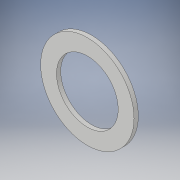
# Autodesk Inventor part: Fixierplatte_Innenring58,2mm
Saved by Autodesk Inventor 2018 (Build 220112000, 112)
## iProperties
Created: 2020-01-21
Part Number: Fixierplatte_Innenring58,2mm
Material: Generisch
Document SubType Name: Modeling
Designer: maxse
Density: 1 g/cm^3
Appearance: Vorgabe
Author: maxse
Autodesk Inventor part; units mm, degrees
ref_plane "YZ Plane" through (0, 0, 0) normal (1, 0, 0) x (0, 1, 0)
ref_plane "XZ Plane" through (0, 0, 0) normal (0, 1, 0) x (-1, 0, 0)
ref_plane "XY Plane" through (0, 0, 0) normal (0, 0, 1) x (1, 0, 0)
sketch "Skizze1" plane through (0, 0, 0) normal (0, 1, 0) x (-1, 0, 0)
  circle A0 centre (0, 0) radius 29.1
  circle A1 centre (0, 0) radius 44
  dimension "d0" = 58.2
  dimension "d1" = 88
  constraints: 2 centre point, 2 coincident
  measures "d0" diameter of A0
  measures "d1" diameter of A1
extrude "Extrusion1" add sketch "Skizze1" along normal blind 4
sketch "Skizze2" plane through (0, 4, 0) normal (0, 1, 0) x (1, 0, 0)
  circle A0 centre (0, 0) radius 29.1 projected
  line L0 (9.4434, -32.7819) -> (9.8648, -32.6469)
  line L1 (9.8648, -32.6469) -> (9.9461, -32.9008)
  spline S0 degree 2 poles (9.9461, -32.9008) (10.0174, -32.7886) (10.1259, -32.6347) (10.2084, -32.5576) knots 0 0 0 1 2 2 2
  spline S1 degree 2 poles (10.2084, -32.5576) (10.2837, -32.4858) (10.4608, -32.3785) (10.5877, -32.3378) knots 0 0 0 1 2 2 2
  spline S2 degree 2 poles (10.5877, -32.3378) (10.793, -32.272) (11.1933, -32.3314) (11.3676, -32.4572) knots 0 0 0 1 2 2 2
  spline S3 degree 2 poles (11.3676, -32.4572) (11.542, -32.583) (11.8328, -33.026) (11.934, -33.342) knots 0 0 0 1 2 2 2
  spline S4 degree 2 poles (11.934, -33.342) (12.0396, -33.6715) (12.0235, -34.2068) (11.9329, -34.4354) knots 0 0 0 1 2 2 2
  spline S5 degree 2 poles (11.9329, -34.4354) (11.8471, -34.6416) (11.5206, -34.9517) (11.3072, -35.0201) knots 0 0 0 1 2 2 2
  spline S6 degree 2 poles (11.3072, -35.0201) (11.1208, -35.0798) (10.8158, -35.0852) (10.6341, -35.0481) knots 0 0 0 1 2 2 2
  line L2 (10.6341, -35.0481) -> (10.9803, -36.1285)
  line L3 (10.9803, -36.1285) -> (10.559, -36.2635)
  line L4 (10.559, -36.2635) -> (9.4434, -32.7819)
  line L5 (10.0595, -33.2546) -> (10.5225, -34.6997)
  spline S7 degree 2 poles (10.5225, -34.6997) (10.7034, -34.7251) (10.9701, -34.7022) (11.1132, -34.6563) knots 0 0 0 1 2 2 2
  spline S8 degree 2 poles (11.1132, -34.6563) (11.4373, -34.5525) (11.6489, -33.9486) (11.5018, -33.4894) knots 0 0 0 1 2 2 2
  spline S9 degree 2 poles (11.5018, -33.4894) (11.3598, -33.0464) (10.9292, -32.6692) (10.6186, -32.7687) knots 0 0 0 1 2 2 2
  spline S10 degree 2 poles (10.6186, -32.7687) (10.4538, -32.8215) (10.1674, -33.0801) (10.0595, -33.2546) knots 0 0 0 1 2 2 2
  spline S11 degree 2 poles (7.7028, -33.158) (8.3153, -33.0121) (9.1523, -33.5386) (9.3035, -34.1732) knots 0 0 0 1 2 2 2
  spline S12 degree 2 poles (9.3035, -34.1732) (9.4521, -34.7967) (8.9744, -35.692) (8.4475, -35.8176) knots 0 0 0 1 2 2 2
  spline S13 degree 2 poles (8.4475, -35.8176) (8.2102, -35.8741) (7.8104, -35.8236) (7.6403, -35.7096) knots 0 0 0 1 2 2 2
  spline S14 degree 2 poles (7.6403, -35.7096) (7.4675, -35.5963) (7.2207, -35.209) (7.1477, -34.9028) knots 0 0 0 1 2 2 2
  line L6 (7.1477, -34.9028) -> (7.0918, -34.6682)
  line L7 (7.0918, -34.6682) -> (8.8603, -34.2467)
  spline S15 degree 2 poles (8.8603, -34.2467) (8.7545, -33.8025) (8.1951, -33.4373) (7.7978, -33.532) knots 0 0 0 1 2 2 2
  spline S16 degree 2 poles (7.7978, -33.532) (7.6571, -33.5655) (7.399, -33.694) (7.3005, -33.77) knots 0 0 0 1 2 2 2
  spline S17 degree 2 poles (7.3005, -33.77) (7.1978, -33.8528) (7.0608, -33.9875) (7.0189, -34.0442) knots 0 0 0 1 2 2 2
  line L8 (7.0189, -34.0442) -> (6.994, -34.0501)
  line L9 (6.994, -34.0501) -> (6.8823, -33.581)
  spline S18 degree 2 poles (6.8823, -33.581) (6.9495, -33.5329) (7.1547, -33.3907) (7.2371, -33.3448) knots 0 0 0 1 2 2 2
  spline S19 degree 2 poles (7.2371, -33.3448) (7.3527, -33.2794) (7.5483, -33.1949) (7.7028, -33.158) knots 0 0 0 1 2 2 2
  spline S20 degree 2 poles (7.5894, -34.8966) (7.6364, -35.0691) (7.7686, -35.3058) (7.858, -35.3749) knots 0 0 0 1 2 2 2
  spline S21 degree 2 poles (7.858, -35.3749) (7.9555, -35.4537) (8.2143, -35.4999) (8.3881, -35.4585) knots 0 0 0 1 2 2 2
  spline S22 degree 2 poles (8.3881, -35.4585) (8.5592, -35.4177) (8.7749, -35.2585) (8.8506, -35.1355) knots 0 0 0 1 2 2 2
  spline S23 degree 2 poles (8.8506, -35.1355) (8.9228, -35.0104) (8.9636, -34.7411) (8.9386, -34.5751) knots 0 0 0 1 2 2 2
  line L10 (8.9386, -34.5751) -> (7.5894, -34.8966)
  spline S24 degree 2 poles (5.6466, -33.566) (5.9068, -33.5226) (6.3806, -33.5873) (6.5419, -33.6409) knots 0 0 0 1 2 2 2
  line L11 (6.5419, -33.6409) -> (6.6236, -34.1304)
  line L12 (6.6236, -34.1304) -> (6.6012, -34.1342)
  spline S25 degree 2 poles (6.6012, -34.1342) (6.5378, -34.0988) (6.369, -34.0177) (6.2333, -33.9799) knots 0 0 0 1 2 2 2
  spline S26 degree 2 poles (6.2333, -33.9799) (6.1153, -33.945) (5.8337, -33.9115) (5.691, -33.9353) knots 0 0 0 1 2 2 2
  spline S27 degree 2 poles (5.691, -33.9353) (5.5875, -33.9526) (5.3576, -34.0398) (5.3082, -34.0883) knots 0 0 0 1 2 2 2
  spline S28 degree 2 poles (5.3082, -34.0883) (5.236, -34.155) (5.1833, -34.2874) (5.2038, -34.4105) knots 0 0 0 1 2 2 2
  spline S29 degree 2 poles (5.2038, -34.4105) (5.2295, -34.5644) (5.424, -34.6959) (5.6483, -34.7131) knots 0 0 0 1 2 2 2
  spline S30 degree 2 poles (5.6483, -34.7131) (5.7355, -34.7186) (6.0134, -34.7298) (6.1332, -34.7414) knots 0 0 0 1 2 2 2
  spline S31 degree 2 poles (6.1332, -34.7414) (6.4442, -34.7786) (6.7726, -35.0919) (6.8151, -35.3465) knots 0 0 0 1 2 2 2
  spline S32 degree 2 poles (6.8151, -35.3465) (6.8739, -35.699) (6.4185, -36.2264) (5.982, -36.2993) knots 0 0 0 1 2 2 2
  spline S33 degree 2 poles (5.982, -36.2993) (5.7666, -36.3352) (5.3124, -36.3018) (5.1506, -36.2454) knots 0 0 0 1 2 2 2
  line L13 (5.1506, -36.2454) -> (5.0726, -35.7782)
  line L14 (5.0726, -35.7782) -> (5.095, -35.7744)
  spline S34 degree 2 poles (5.095, -35.7744) (5.2853, -35.8807) (5.7194, -35.9664) (5.9293, -35.9314) knots 0 0 0 1 2 2 2
  spline S35 degree 2 poles (5.9293, -35.9314) (6.1447, -35.8954) (6.4109, -35.6641) (6.3805, -35.4823) knots 0 0 0 1 2 2 2
  spline S36 degree 2 poles (6.3805, -35.4823) (6.353, -35.3172) (6.1501, -35.1872) (5.9459, -35.1695) knots 0 0 0 1 2 2 2
  spline S37 degree 2 poles (5.9459, -35.1695) (5.8465, -35.1602) (5.5975, -35.15) (5.4609, -35.1411) knots 0 0 0 1 2 2 2
  spline S38 degree 2 poles (5.4609, -35.1411) (5.1634, -35.116) (4.8169, -34.8317) (4.7688, -34.5435) knots 0 0 0 1 2 2 2
  spline S39 degree 2 poles (4.7688, -34.5435) (4.7408, -34.3757) (4.8228, -34.0572) (4.9333, -33.9266) knots 0 0 0 1 2 2 2
  spline S40 degree 2 poles (4.9333, -33.9266) (5.0512, -33.789) (5.3808, -33.6104) (5.6466, -33.566) knots 0 0 0 1 2 2 2
  line L15 (3.7868, -33.8898) -> (4.2262, -33.8378)
  line L16 (4.2262, -33.8378) -> (4.5348, -36.446)
  line L17 (4.5348, -36.446) -> (4.0954, -36.498)
  line L18 (4.0954, -36.498) -> (3.7868, -33.8898)
  line L19 (4.1158, -36.9355) -> (4.6143, -36.8765)
  line L20 (4.6143, -36.8765) -> (4.6683, -37.3328)
  line L21 (4.6683, -37.3328) -> (4.1697, -37.3918)
  line L22 (4.1697, -37.3918) -> (4.1158, -36.9355)
  spline S41 degree 2 poles (3.0227, -33.5568) (2.9762, -33.5398) (2.7996, -33.4884) (2.6876, -33.4698) knots 0 0 0 1 2 2 2
  spline S42 degree 2 poles (2.6876, -33.4698) (2.5639, -33.4463) (2.355, -33.4225) (2.2333, -33.4301) knots 0 0 0 1 2 2 2
  spline S43 degree 2 poles (2.2333, -33.4301) (2.0294, -33.4429) (1.7531, -33.5682) (1.6799, -33.6695) knots 0 0 0 1 2 2 2
  spline S44 degree 2 poles (1.6799, -33.6695) (1.6095, -33.7705) (1.5659, -34.0262) (1.576, -34.1875) knots 0 0 0 1 2 2 2
  line L23 (1.576, -34.1875) -> (1.5904, -34.4168)
  spline S45 degree 2 poles (1.5904, -34.4168) (1.7589, -34.2499) (2.0922, -34.0813) (2.3498, -34.0651) knots 0 0 0 1 2 2 2
  spline S46 degree 2 poles (2.3498, -34.0651) (2.7971, -34.037) (3.3681, -34.6691) (3.4074, -35.2947) knots 0 0 0 1 2 2 2
  spline S47 degree 2 poles (3.4074, -35.2947) (3.4278, -35.6202) (3.2754, -36.1356) (3.1337, -36.3235) knots 0 0 0 1 2 2 2
  spline S48 degree 2 poles (3.1337, -36.3235) (2.997, -36.4998) (2.6038, -36.7092) (2.3886, -36.7227) knots 0 0 0 1 2 2 2
  spline S49 degree 2 poles (2.3886, -36.7227) (2.1848, -36.7354) (1.8815, -36.6578) (1.726, -36.5795) knots 0 0 0 1 2 2 2
  line L24 (1.726, -36.5795) -> (1.7075, -36.6915)
  line L25 (1.7075, -36.6915) -> (1.2913, -36.7176)
  line L26 (1.2913, -36.7176) -> (1.1457, -34.3964)
  spline S50 degree 2 poles (1.1457, -34.3964) (1.1038, -33.7283) (1.6451, -33.0692) (2.2424, -33.0317) knots 0 0 0 1 2 2 2
  spline S51 degree 2 poles (2.2424, -33.0317) (2.4349, -33.0196) (2.8407, -33.0567) (3.0166, -33.0968) knots 0 0 0 1 2 2 2
  line L27 (3.0166, -33.0968) -> (3.0454, -33.5554)
  line L28 (3.0454, -33.5554) -> (3.0227, -33.5568)
  line L29 (1.6131, -34.7791) -> (1.7035, -36.22)
  spline S52 degree 2 poles (1.7035, -36.22) (1.8726, -36.289) (2.1543, -36.3395) (2.293, -36.3308) knots 0 0 0 1 2 2 2
  spline S53 degree 2 poles (2.293, -36.3308) (2.627, -36.3098) (2.9811, -35.7931) (2.9522, -35.3317) knots 0 0 0 1 2 2 2
  spline S54 degree 2 poles (2.9522, -35.3317) (2.9248, -34.8958) (2.6047, -34.4583) (2.2763, -34.4789) knots 0 0 0 1 2 2 2
  spline S55 degree 2 poles (2.2763, -34.4789) (2.1036, -34.4898) (1.7498, -34.6484) (1.6131, -34.7791) knots 0 0 0 1 2 2 2
  line L30 (-1.5751, -34.0795) -> (-1.1327, -34.0864)
  line L31 (-1.1327, -34.0864) -> (-1.1562, -35.5838)
  spline S56 degree 2 poles (-1.1562, -35.5838) (-1.159, -35.7653) (-1.1299, -36.0778) (-1.0803, -36.1722) knots 0 0 0 1 2 2 2
  spline S57 degree 2 poles (-1.0803, -36.1722) (-1.028, -36.2723) (-0.8367, -36.3717) (-0.6722, -36.3743) knots 0 0 0 1 2 2 2
  spline S58 degree 2 poles (-0.6722, -36.3743) (-0.5077, -36.3769) (-0.1561, -36.2065) (0.0134, -36.0674) knots 0 0 0 1 2 2 2
  line L32 (0.0134, -36.0674) -> (0.0442, -34.1049)
  line L33 (0.0442, -34.1049) -> (0.4866, -34.1118)
  line L34 (0.4866, -34.1118) -> (0.4454, -36.7379)
  line L35 (0.4454, -36.7379) -> (0.003, -36.731)
  line L36 (0.003, -36.731) -> (0.0076, -36.4389)
  spline S59 degree 2 poles (0.0076, -36.4389) (-0.1937, -36.6144) (-0.5795, -36.7956) (-0.795, -36.7922) knots 0 0 0 1 2 2 2
  spline S60 degree 2 poles (-0.795, -36.7922) (-1.1807, -36.7862) (-1.6095, -36.2689) (-1.6019, -35.7839) knots 0 0 0 1 2 2 2
  line L37 (-1.6019, -35.7839) -> (-1.5751, -34.0795)
  spline S61 degree 2 poles (-3.3246, -33.8783) (-2.6976, -33.9362) (-2.0735, -34.7031) (-2.1335, -35.3527) knots 0 0 0 1 2 2 2
  spline S62 degree 2 poles (-2.1335, -35.3527) (-2.1924, -35.9909) (-2.9317, -36.686) (-3.4711, -36.6362) knots 0 0 0 1 2 2 2
  spline S63 degree 2 poles (-3.4711, -36.6362) (-3.714, -36.6138) (-4.0766, -36.4378) (-4.2012, -36.2754) knots 0 0 0 1 2 2 2
  spline S64 degree 2 poles (-4.2012, -36.2754) (-4.3286, -36.1126) (-4.4383, -35.6667) (-4.4094, -35.3532) knots 0 0 0 1 2 2 2
  line L38 (-4.4094, -35.3532) -> (-4.3872, -35.1131)
  line L39 (-4.3872, -35.1131) -> (-2.5768, -35.2804)
  spline S65 degree 2 poles (-2.5768, -35.2804) (-2.5348, -34.8257) (-2.9478, -34.3004) (-3.3545, -34.2629) knots 0 0 0 1 2 2 2
  spline S66 degree 2 poles (-3.3545, -34.2629) (-3.4985, -34.2496) (-3.7841, -34.2887) (-3.9018, -34.3291) knots 0 0 0 1 2 2 2
  spline S67 degree 2 poles (-3.9018, -34.3291) (-4.0256, -34.3746) (-4.1985, -34.4583) (-4.2564, -34.4986) knots 0 0 0 1 2 2 2
  line L40 (-4.2564, -34.4986) -> (-4.2818, -34.4962)
  line L41 (-4.2818, -34.4962) -> (-4.2374, -34.0161)
  spline S68 degree 2 poles (-4.2374, -34.0161) (-4.1583, -33.9921) (-3.9184, -33.9231) (-3.8257, -33.906) knots 0 0 0 1 2 2 2
  spline S69 degree 2 poles (-3.8257, -33.906) (-3.6952, -33.8811) (-3.4828, -33.8636) (-3.3246, -33.8783) knots 0 0 0 1 2 2 2
  spline S70 degree 2 poles (-3.989, -35.4889) (-3.9997, -35.6673) (-3.9503, -35.934) (-3.8878, -36.028) knots 0 0 0 1 2 2 2
  spline S71 degree 2 poles (-3.8878, -36.028) (-3.8207, -36.1339) (-3.5903, -36.2606) (-3.4123, -36.277) knots 0 0 0 1 2 2 2
  spline S72 degree 2 poles (-3.4123, -36.277) (-3.2372, -36.2932) (-2.9819, -36.2114) (-2.8708, -36.1191) knots 0 0 0 1 2 2 2
  spline S73 degree 2 poles (-2.8708, -36.1191) (-2.7623, -36.0238) (-2.6374, -35.7818) (-2.6079, -35.6165) knots 0 0 0 1 2 2 2
  line L42 (-2.6079, -35.6165) -> (-3.989, -35.4889)
  line L43 (-6.7049, -33.4496) -> (-6.2687, -33.5237)
  line L44 (-6.2687, -33.5237) -> (-6.3133, -33.7865)
  spline S74 degree 2 poles (-6.3133, -33.7865) (-6.1984, -33.7197) (-6.0312, -33.633) (-5.9225, -33.6026) knots 0 0 0 1 2 2 2
  spline S75 degree 2 poles (-5.9225, -33.6026) (-5.8226, -33.5735) (-5.616, -33.5597) (-5.4846, -33.582) knots 0 0 0 1 2 2 2
  spline S76 degree 2 poles (-5.4846, -33.582) (-5.2721, -33.6181) (-4.9441, -33.8551) (-4.8472, -34.047) knots 0 0 0 1 2 2 2
  spline S77 degree 2 poles (-4.8472, -34.047) (-4.7503, -34.2389) (-4.696, -34.766) (-4.7516, -35.0932) knots 0 0 0 1 2 2 2
  spline S78 degree 2 poles (-4.7516, -35.0932) (-4.8095, -35.4343) (-5.0702, -35.9021) (-5.2558, -36.0634) knots 0 0 0 1 2 2 2
  spline S79 degree 2 poles (-5.2558, -36.0634) (-5.4269, -36.2069) (-5.8595, -36.332) (-6.0804, -36.2944) knots 0 0 0 1 2 2 2
  spline S80 degree 2 poles (-6.0804, -36.2944) (-6.2734, -36.2617) (-6.5467, -36.1261) (-6.6909, -36.0095) knots 0 0 0 1 2 2 2
  line L45 (-6.6909, -36.0095) -> (-6.8808, -37.128)
  line L46 (-6.8808, -37.128) -> (-7.317, -37.054)
  line L47 (-7.317, -37.054) -> (-6.7049, -33.4496)
  line L48 (-6.3755, -34.1528) -> (-6.6296, -35.6488)
  spline S81 degree 2 poles (-6.6296, -35.6488) (-6.4807, -35.7547) (-6.2334, -35.8571) (-6.0852, -35.8822) knots 0 0 0 1 2 2 2
  spline S82 degree 2 poles (-6.0852, -35.8822) (-5.7497, -35.9392) (-5.2839, -35.5005) (-5.2032, -35.0251) knots 0 0 0 1 2 2 2
  spline S83 degree 2 poles (-5.2032, -35.0251) (-5.1253, -34.5665) (-5.334, -34.0334) (-5.6555, -33.9788) knots 0 0 0 1 2 2 2
  spline S84 degree 2 poles (-5.6555, -33.9788) (-5.8261, -33.9498) (-6.1994, -34.0475) (-6.3755, -34.1528) knots 0 0 0 1 2 2 2
  spline S85 degree 2 poles (-11.2896, -33.6315) (-11.1053, -33.0145) (-10.2826, -32.4404) (-9.8314, -32.5751) knots 0 0 0 1 2 2 2
  spline S86 degree 2 poles (-9.8314, -32.5751) (-9.6276, -32.636) (-9.3669, -32.8234) (-9.2515, -32.9526) knots 0 0 0 1 2 2 2
  line L49 (-9.2515, -32.9526) -> (-9.1894, -32.8439)
  line L50 (-9.1894, -32.8439) -> (-8.7927, -32.9624)
  line L51 (-8.7927, -32.9624) -> (-9.8391, -36.4654)
  line L52 (-9.8391, -36.4654) -> (-10.263, -36.3388)
  line L53 (-10.263, -36.3388) -> (-9.8896, -35.0887)
  spline S87 degree 2 poles (-9.8896, -35.0887) (-10.093, -35.1848) (-10.5221, -35.2638) (-10.7585, -35.1932) knots 0 0 0 1 2 2 2
  spline S88 degree 2 poles (-10.7585, -35.1932) (-11.1852, -35.0657) (-11.4706, -34.2375) (-11.2896, -33.6315) knots 0 0 0 1 2 2 2
  spline S89 degree 2 poles (-10.8423, -33.7295) (-10.9771, -34.1807) (-10.8422, -34.7301) (-10.5378, -34.821) knots 0 0 0 1 2 2 2
  spline S90 degree 2 poles (-10.5378, -34.821) (-10.3666, -34.8722) (-9.9646, -34.8146) (-9.7832, -34.7327) knots 0 0 0 1 2 2 2
  line L54 (-9.7832, -34.7327) -> (-9.3522, -33.2896)
  spline S91 degree 2 poles (-9.3522, -33.2896) (-9.489, -33.1629) (-9.7168, -33.0238) (-9.8635, -32.9799) knots 0 0 0 1 2 2 2
  spline S92 degree 2 poles (-9.8635, -32.9799) (-10.1869, -32.8833) (-10.6937, -33.2322) (-10.8423, -33.7295) knots 0 0 0 1 2 2 2
  line L55 (-14.1952, -33.8929) -> (-11.5948, -31.0386)
  line L56 (-11.5948, -31.0386) -> (-11.1522, -31.2075)
  line L57 (-11.1522, -31.2075) -> (-11.9823, -32.0626)
  line L58 (-11.9823, -32.0626) -> (-11.9824, -34.7369)
  line L59 (-11.9824, -34.7369) -> (-12.4276, -34.5671)
  line L60 (-12.4276, -34.5671) -> (-12.4047, -32.4934)
  line L61 (-12.4047, -32.4934) -> (-13.7659, -34.0566)
  line L62 (-13.7659, -34.0566) -> (-14.1952, -33.8929)
  line L63 (18.0086, 34.7463) -> (16.5324, 31.5728)
  line L64 (16.5324, 31.5728) -> (15.9011, 31.8665)
  line L65 (15.9011, 31.8665) -> (16.1941, 34.4634)
  spline S93 degree 2 poles (16.1941, 34.4634) (16.2363, 34.8263) (16.26, 35.0036) knots 0 0 0 1 1 1
  spline S94 degree 2 poles (16.26, 35.0036) (16.1269, 34.8566) (15.8544, 34.5744) knots 0 0 0 1 1 1
  line L66 (15.8544, 34.5744) -> (14.0652, 32.7204)
  line L67 (14.0652, 32.7204) -> (13.5016, 32.9826)
  line L68 (13.5016, 32.9826) -> (14.9778, 36.1561)
  line L69 (14.9778, 36.1561) -> (15.3817, 35.9682)
  line L70 (15.3817, 35.9682) -> (14.1463, 33.3123)
  line L71 (14.1463, 33.3123) -> (16.3081, 35.5372)
  line L72 (16.3081, 35.5372) -> (16.6855, 35.3617)
  line L73 (16.6855, 35.3617) -> (16.3479, 32.2324)
  line L74 (16.3479, 32.2324) -> (17.6046, 34.9342)
  line L75 (17.6046, 34.9342) -> (18.0086, 34.7463)
  spline S95 degree 2 poles (12.6685, 36.6659) (12.9634, 36.7745) (13.4336, 36.7796) (13.6718, 36.693) knots 0 0 0 1 2 2 2
  spline S96 degree 2 poles (13.6718, 36.693) (14.0654, 36.5499) (14.3472, 36.0132) (14.2388, 35.7149) knots 0 0 0 1 2 2 2
  spline S97 degree 2 poles (14.2388, 35.7149) (14.175, 35.5394) (13.9098, 35.3094) (13.5902, 35.2268) (13.4118, 35.2434) knots 0 0 0 1 2 3 3 3
  spline S98 degree 2 poles (13.4118, 35.2434) (13.2821, 35.2536) (13.0305, 35.311) knots 0 0 0 1 1 1
  spline S99 degree 2 poles (13.0305, 35.311) (12.5206, 35.431) (12.2608, 35.4346) knots 0 0 0 1 1 1
  spline S100 degree 2 poles (12.2608, 35.4346) (12.2282, 35.3528) (12.22, 35.3303) knots 0 0 0 1 1 1
  spline S101 degree 2 poles (12.22, 35.3303) (12.1298, 35.082) (12.2087, 34.9398) knots 0 0 0 1 1 1
  spline S102 degree 2 poles (12.2087, 34.9398) (12.3115, 34.7464) (12.6174, 34.6352) knots 0 0 0 1 1 1
  spline S103 degree 2 poles (12.6174, 34.6352) (12.9007, 34.5322) (13.2444, 34.6344) (13.4016, 34.8639) knots 0 0 0 1 2 2 2
  line L76 (13.4016, 34.8639) -> (13.7786, 34.6673)
  spline S104 degree 2 poles (13.7786, 34.6673) (13.6339, 34.4332) (13.2718, 34.21) (12.7444, 34.2115) (12.4385, 34.3227) knots 0 0 0 1 2 3 3 3
  spline S105 degree 2 poles (12.4385, 34.3227) (12.1326, 34.4338) (11.8035, 34.7153) (11.7022, 34.999) (11.7273, 35.1772) knots 0 0 0 1 2 3 3 3
  spline S106 degree 2 poles (11.7273, 35.1772) (11.7455, 35.2898) (11.843, 35.5581) knots 0 0 0 1 1 1
  line L77 (11.843, 35.5581) -> (12.0389, 36.0972)
  spline S107 degree 2 poles (12.0389, 36.0972) (12.243, 36.6588) (12.2988, 36.9763) (12.2737, 37.1415) knots 0 0 0 1 2 2 2
  line L78 (12.2737, 37.1415) -> (12.6949, 36.9884)
  spline S108 degree 2 poles (12.6949, 36.9884) (12.712, 36.8403) (12.6685, 36.6659) knots 0 0 0 1 1 1
  spline S109 degree 2 poles (12.3731, 35.7515) (12.6265, 35.7615) (13.0881, 35.6648) knots 0 0 0 1 1 1
  spline S110 degree 2 poles (13.0881, 35.6648) (13.3515, 35.6087) (13.5899, 35.6243) (13.7656, 35.7563) (13.8039, 35.8616) knots 0 0 0 1 2 3 3 3
  spline S111 degree 2 poles (13.8039, 35.8616) (13.8622, 36.022) (13.6974, 36.3261) (13.4617, 36.4117) knots 0 0 0 1 2 2 2
  spline S112 degree 2 poles (13.4617, 36.4117) (13.2285, 36.4965) (12.7912, 36.4255) (12.6412, 36.2785) knots 0 0 0 1 2 2 2
  spline S113 degree 2 poles (12.6412, 36.2785) (12.5259, 36.1643) (12.4293, 35.8985) knots 0 0 0 1 1 1
  line L79 (12.4293, 35.8985) -> (12.3731, 35.7515)
  line L80 (12.0434, 37.218) -> (10.7859, 36.2164)
  line L81 (10.7859, 36.2164) -> (11.2694, 34.801)
  line L82 (11.2694, 34.801) -> (10.7571, 34.9497)
  line L83 (10.7571, 34.9497) -> (10.5438, 35.6311)
  spline S114 degree 2 poles (10.5438, 35.6311) (10.483, 35.8238) (10.4502, 35.95) knots 0 0 0 1 1 1
  spline S115 degree 2 poles (10.4502, 35.95) (10.3061, 35.8362) (10.1899, 35.7422) knots 0 0 0 1 1 1
  line L84 (10.1899, 35.7422) -> (9.6119, 35.2822)
  line L85 (9.6119, 35.2822) -> (9.1149, 35.4265)
  line L86 (9.1149, 35.4265) -> (10.279, 36.3552)
  line L87 (10.279, 36.3552) -> (9.7633, 37.88)
  line L88 (9.7633, 37.88) -> (10.2706, 37.7327)
  line L89 (10.2706, 37.7327) -> (10.554, 36.8337)
  line L90 (10.554, 36.8337) -> (10.6183, 36.6151)
  line L91 (10.6183, 36.6151) -> (11.5439, 37.363)
  line L92 (11.5439, 37.363) -> (12.0434, 37.218)
  line L93 (7.9981, 37.1493) -> (7.5608, 37.1886)
  spline S116 degree 2 poles (7.5608, 37.1886) (7.5752, 37.4543) (7.4104, 37.8247) (6.9763, 38.1127) (6.6821, 38.1647) knots 0 0 0 1 2 3 3 3
  spline S117 degree 2 poles (6.6821, 38.1647) (6.4221, 38.2106) (5.9927, 38.1267) (5.7505, 37.8904) (5.7222, 37.7302) knots 0 0 0 1 2 3 3 3
  spline S118 degree 2 poles (5.7222, 37.7302) (5.6934, 37.5673) (5.8373, 37.2927) (6.0409, 37.1727) knots 0 0 0 1 2 2 2
  spline S119 degree 2 poles (6.0409, 37.1727) (6.1704, 37.0929) (7.0836, 36.6959) (7.2573, 36.5596) knots 0 0 0 1 2 2 2
  spline S120 degree 2 poles (7.2573, 36.5596) (7.4815, 36.3872) (7.6554, 35.961) (7.6136, 35.7245) knots 0 0 0 1 2 2 2
  spline S121 degree 2 poles (7.6136, 35.7245) (7.5672, 35.4618) (7.1905, 35.0625) (6.5787, 34.9267) (6.2293, 34.9885) knots 0 0 0 1 2 3 3 3
  spline S122 degree 2 poles (6.2293, 34.9885) (5.8458, 35.0562) (5.3036, 35.4067) (5.0706, 35.9436) (5.1135, 36.2475) knots 0 0 0 1 2 3 3 3
  line L94 (5.1135, 36.2475) -> (5.5556, 36.2046)
  spline S123 degree 2 poles (5.5556, 36.2046) (5.5318, 35.8702) (5.8826, 35.4642) (6.2819, 35.3937) knots 0 0 0 1 2 2 2
  spline S124 degree 2 poles (6.2819, 35.3937) (6.697, 35.3203) (7.1317, 35.5577) (7.1693, 35.7705) knots 0 0 0 1 2 2 2
  spline S125 degree 2 poles (7.1693, 35.7705) (7.2023, 35.957) (7.0897, 36.1016) knots 0 0 0 1 1 1
  spline S126 degree 2 poles (7.0897, 36.1016) (6.9766, 36.2434) (5.9047, 36.6929) (5.7138, 36.8241) knots 0 0 0 1 2 2 2
  spline S127 degree 2 poles (5.7138, 36.8241) (5.439, 37.0163) (5.2278, 37.4925) (5.2765, 37.7683) knots 0 0 0 1 2 2 2
  spline S128 degree 2 poles (5.2765, 37.7683) (5.3253, 38.0441) (5.7264, 38.4744) (6.3653, 38.6406) (6.7331, 38.5756) knots 0 0 0 1 2 3 3 3
  spline S129 degree 2 poles (6.7331, 38.5756) (7.2033, 38.4925) (7.7855, 38.1079) (8.0488, 37.4979) (7.9981, 37.1493) knots 0 0 0 1 2 3 3 3
  line L95 (3.0679, 38.1643) -> (2.63, 38.2638)
  spline S130 degree 2 poles (2.63, 38.2638) (2.7745, 38.6409) (3.3822, 39.0125) (3.8202, 38.9692) knots 0 0 0 1 2 2 2
  spline S131 degree 2 poles (3.8202, 38.9692) (4.375, 38.9144) (4.9554, 38.1682) (4.8949, 37.5549) knots 0 0 0 1 2 2 2
  spline S132 degree 2 poles (4.8949, 37.5549) (4.832, 36.9178) (4.1068, 36.279) (3.5838, 36.3307) knots 0 0 0 1 2 2 2
  spline S133 degree 2 poles (3.5838, 36.3307) (3.0794, 36.3805) (2.5051, 37.1342) (2.5667, 37.7581) knots 0 0 0 1 2 2 2
  spline S134 degree 2 poles (2.5667, 37.7581) (2.5703, 37.7952) (2.5806, 37.8719) knots 0 0 0 1 1 1
  line L96 (2.5806, 37.8719) -> (4.4628, 37.6861)
  spline S135 degree 2 poles (4.4628, 37.6861) (4.4801, 38.1052) (4.1015, 38.5876) (3.7856, 38.6188) knots 0 0 0 1 2 2 2
  spline S136 degree 2 poles (3.7856, 38.6188) (3.5493, 38.6421) (3.1928, 38.4254) (3.0679, 38.1643) knots 0 0 0 1 2 2 2
  line L97 (4.4043, 37.338) -> (2.9947, 37.4772)
  spline S137 degree 2 poles (2.9947, 37.4772) (2.9924, 37.1558) (3.1091, 36.9807) knots 0 0 0 1 1 1
  spline S138 degree 2 poles (3.1091, 36.9807) (3.2892, 36.7136) (3.6157, 36.6814) knots 0 0 0 1 1 1
  spline S139 degree 2 poles (3.6157, 36.6814) (3.9104, 36.6523) (4.3503, 37.0082) (4.4043, 37.338) knots 0 0 0 1 2 2 2
  line L98 (2.3158, 38.2874) -> (1.8897, 38.2345)
  spline S140 degree 2 poles (1.8897, 38.2345) (1.8634, 38.4916) (1.5442, 38.7742) (1.2483, 38.7838) knots 0 0 0 1 2 2 2
  spline S141 degree 2 poles (1.2483, 38.7838) (0.9523, 38.7934) (0.6565, 38.5601) (0.6512, 38.3975) knots 0 0 0 1 2 2 2
  spline S142 degree 2 poles (0.6512, 38.3975) (0.6465, 38.2535) (0.7717, 38.164) knots 0 0 0 1 1 1
  spline S143 degree 2 poles (0.7717, 38.164) (0.8579, 38.1052) (1.207, 38.0058) knots 0 0 0 1 1 1
  spline S144 degree 2 poles (1.207, 38.0058) (1.6751, 37.8705) (2.0347, 37.6853) (2.214, 37.3699) (2.208, 37.1859) knots 0 0 0 1 2 3 3 3
  spline S145 degree 2 poles (2.208, 37.1859) (2.2025, 37.0153) (2.0385, 36.7323) (1.9021, 36.6407) knots 0 0 0 1 2 2 2
  spline S146 degree 2 poles (1.9021, 36.6407) (1.7984, 36.5693) (1.4484, 36.4792) (1.2485, 36.4857) knots 0 0 0 1 2 2 2
  spline S147 degree 2 poles (1.2485, 36.4857) (0.9499, 36.4954) (0.5049, 36.6833) (0.2984, 36.9836) (0.2664, 37.2302) knots 0 0 0 1 2 3 3 3
  line L99 (0.2664, 37.2302) -> (0.6895, 37.2725)
  spline S148 degree 2 poles (0.6895, 37.2725) (0.7124, 37.0743) (0.9799, 36.8467) (1.2306, 36.8386) knots 0 0 0 1 2 2 2
  spline S149 degree 2 poles (1.2306, 36.8386) (1.5265, 36.829) (1.7862, 37.0181) (1.7904, 37.1488) knots 0 0 0 1 2 2 2
  spline S150 degree 2 poles (1.7904, 37.1488) (1.7931, 37.2314) (1.742, 37.2998) knots 0 0 0 1 1 1
  spline S151 degree 2 poles (1.742, 37.2998) (1.6936, 37.3708) (1.5804, 37.4198) knots 0 0 0 1 1 1
  spline S152 degree 2 poles (1.5804, 37.4198) (1.5172, 37.4459) (1.2054, 37.5441) knots 0 0 0 1 1 1
  spline S153 degree 2 poles (1.2054, 37.5441) (0.7533, 37.6788) (0.3957, 37.8452) (0.2, 38.1479) (0.2072, 38.3692) knots 0 0 0 1 2 3 3 3
  spline S154 degree 2 poles (0.2072, 38.3692) (0.2141, 38.5825) (0.477, 38.9529) (0.9584, 39.1455) (1.257, 39.1358) knots 0 0 0 1 2 3 3 3
  spline S155 degree 2 poles (1.257, 39.1358) (1.7503, 39.1198) (2.2569, 38.6924) (2.3158, 38.2874) knots 0 0 0 1 2 2 2
  line L100 (-0.0818, 38.3573) -> (-0.5038, 38.2779)
  spline S156 degree 2 poles (-0.5038, 38.2779) (-0.5461, 38.5328) (-0.8823, 38.7949) (-1.1783, 38.786) knots 0 0 0 1 2 2 2
  spline S157 degree 2 poles (-1.1783, 38.786) (-1.4743, 38.7771) (-1.7549, 38.5257) (-1.75, 38.3631) knots 0 0 0 1 2 2 2
  spline S158 degree 2 poles (-1.75, 38.3631) (-1.7457, 38.2191) (-1.6151, 38.1376) knots 0 0 0 1 1 1
  spline S159 degree 2 poles (-1.6151, 38.1376) (-1.5254, 38.0843) (-1.1708, 38.0069) knots 0 0 0 1 1 1
  spline S160 degree 2 poles (-1.1708, 38.0069) (-0.6952, 37.9011) (-0.3247, 37.7388) (-0.1261, 37.4352) (-0.1205, 37.2512) knots 0 0 0 1 2 3 3 3
  spline S161 degree 2 poles (-0.1205, 37.2512) (-0.1154, 37.0806) (-0.2614, 36.7879) (-0.3918, 36.6879) knots 0 0 0 1 2 2 2
  spline S162 degree 2 poles (-0.3918, 36.6879) (-0.4909, 36.6102) (-0.8345, 36.4984) (-1.0344, 36.4924) knots 0 0 0 1 2 2 2
  spline S163 degree 2 poles (-1.0344, 36.4924) (-1.3331, 36.4834) (-1.7889, 36.6432) (-2.0138, 36.93) (-2.0612, 37.1741) knots 0 0 0 1 2 3 3 3
  line L101 (-2.0612, 37.1741) -> (-1.6415, 37.2428)
  spline S164 degree 2 poles (-1.6415, 37.2428) (-1.6063, 37.0463) (-1.325, 36.8359) (-1.0744, 36.8435) knots 0 0 0 1 2 2 2
  spline S165 degree 2 poles (-1.0744, 36.8435) (-0.7784, 36.8524) (-0.531, 37.0574) (-0.535, 37.188) knots 0 0 0 1 2 2 2
  spline S166 degree 2 poles (-0.535, 37.188) (-0.5375, 37.2707) (-0.5928, 37.3357) knots 0 0 0 1 1 1
  spline S167 degree 2 poles (-0.5928, 37.3357) (-0.6455, 37.4036) (-0.7616, 37.4454) knots 0 0 0 1 1 1
  spline S168 degree 2 poles (-0.7616, 37.4454) (-0.8263, 37.4675) (-1.1436, 37.546) knots 0 0 0 1 1 1
  spline S169 degree 2 poles (-1.1436, 37.546) (-1.6032, 37.6523) (-1.9705, 37.796) (-2.1847, 38.0858) (-2.1914, 38.3071) knots 0 0 0 1 2 3 3 3
  spline S170 degree 2 poles (-2.1914, 38.3071) (-2.1978, 38.5204) (-1.9586, 38.9066) (-1.4902, 39.1289) (-1.1916, 39.1379) knots 0 0 0 1 2 3 3 3
  spline S171 degree 2 poles (-1.1916, 39.1379) (-0.6983, 39.1528) (-0.1659, 38.7578) (-0.0818, 38.3573) knots 0 0 0 1 2 2 2
  line L102 (-4.3694, 38.0372) -> (-4.8182, 38.0502)
  spline S172 degree 2 poles (-4.8182, 38.0502) (-4.7494, 38.4482) (-4.225, 38.9302) (-3.7869, 38.9725) knots 0 0 0 1 2 2 2
  spline S173 degree 2 poles (-3.7869, 38.9725) (-3.2319, 39.026) (-2.5182, 38.4061) (-2.459, 37.7927) knots 0 0 0 1 2 2 2
  spline S174 degree 2 poles (-2.459, 37.7927) (-2.3976, 37.1554) (-2.9856, 36.3885) (-3.5087, 36.338) knots 0 0 0 1 2 2 2
  spline S175 degree 2 poles (-3.5087, 36.338) (-4.0132, 36.2894) (-4.7224, 36.9178) (-4.7826, 37.5418) knots 0 0 0 1 2 2 2
  spline S176 degree 2 poles (-4.7826, 37.5418) (-4.7862, 37.579) (-4.7909, 37.6562) knots 0 0 0 1 1 1
  line L103 (-4.7909, 37.6562) -> (-2.9083, 37.8378)
  spline S177 degree 2 poles (-2.9083, 37.8378) (-2.9724, 38.2524) (-3.4371, 38.6524) (-3.7531, 38.622) knots 0 0 0 1 2 2 2
  spline S178 degree 2 poles (-3.7531, 38.622) (-3.9894, 38.5992) (-4.2973, 38.3176) (-4.3694, 38.0372) knots 0 0 0 1 2 2 2
  line L104 (-2.8984, 37.485) -> (-4.3084, 37.349)
  spline S179 degree 2 poles (-4.3084, 37.349) (-4.2484, 37.0332) (-4.1, 36.884) knots 0 0 0 1 1 1
  spline S180 degree 2 poles (-4.1, 36.884) (-3.8718, 36.6568) (-3.5452, 36.6883) knots 0 0 0 1 1 1
  spline S181 degree 2 poles (-3.5452, 36.6883) (-3.2504, 36.7167) (-2.8876, 37.151) (-2.8984, 37.485) knots 0 0 0 1 2 2 2
  line L105 (-5.4128, 38.7242) -> (-4.9078, 35.2608)
  line L106 (-4.9078, 35.2608) -> (-5.3328, 35.1989)
  line L107 (-5.3328, 35.1989) -> (-5.8378, 38.6622)
  line L108 (-5.8378, 38.6622) -> (-5.4128, 38.7242)
  line L109 (-6.5018, 38.5937) -> (-5.9712, 36.1129)
  line L110 (-5.9712, 36.1129) -> (-6.3468, 36.0325)
  line L111 (-6.3468, 36.0325) -> (-6.4216, 36.3821)
  spline S182 degree 2 poles (-6.4216, 36.3821) (-6.4999, 36.1744) (-6.8386, 35.87) (-7.0864, 35.817) knots 0 0 0 1 2 2 2
  spline S183 degree 2 poles (-7.0864, 35.817) (-7.3629, 35.7579) (-7.7642, 35.9121) (-7.8813, 36.1026) knots 0 0 0 1 2 2 2
  spline S184 degree 2 poles (-7.8813, 36.1026) (-8.0829, 35.6039) (-8.5551, 35.5029) knots 0 0 0 1 1 1
  spline S185 degree 2 poles (-8.5551, 35.5029) (-8.9229, 35.4242) (-9.4096, 35.7484) (-9.5006, 36.1737) knots 0 0 0 1 2 2 2
  line L112 (-9.5006, 36.1737) -> (-9.8644, 37.8745)
  line L113 (-9.8644, 37.8745) -> (-9.4444, 37.9643)
  line L114 (-9.4444, 37.9643) -> (-9.1102, 36.4017)
  spline S186 degree 2 poles (-9.1102, 36.4017) (-9.0566, 36.1513) (-8.9257, 35.9474) (-8.6828, 35.8575) (-8.5393, 35.8882) knots 0 0 0 1 2 3 3 3
  spline S187 degree 2 poles (-8.5393, 35.8882) (-8.2758, 35.9446) (-8.0057, 36.3652) (-8.0877, 36.7486) knots 0 0 0 1 2 2 2
  line L115 (-8.0877, 36.7486) -> (-8.3957, 38.1886)
  line L116 (-8.3957, 38.1886) -> (-7.9757, 38.2785)
  line L117 (-7.9757, 38.2785) -> (-7.6314, 36.6689)
  spline S188 degree 2 poles (-7.6314, 36.6689) (-7.5712, 36.3872) (-7.3054, 36.1521) (-7.0706, 36.2023) knots 0 0 0 1 2 2 2
  spline S189 degree 2 poles (-7.0706, 36.2023) (-6.8932, 36.2403) (-6.6334, 36.4923) (-6.5742, 36.8787) (-6.6467, 37.2178) knots 0 0 0 1 2 3 3 3
  line L118 (-6.6467, 37.2178) -> (-6.9218, 38.5039)
  line L119 (-6.9218, 38.5039) -> (-6.5018, 38.5937)
  spline S190 degree 2 poles (-11.9604, 36.903) (-11.7903, 37.1672) (-11.4179, 37.4544) (-11.1756, 37.5287) knots 0 0 0 1 2 2 2
  spline S191 degree 2 poles (-11.1756, 37.5287) (-10.7752, 37.6514) (-10.2271, 37.3926) (-10.134, 37.0891) knots 0 0 0 1 2 2 2
  spline S192 degree 2 poles (-10.134, 37.0891) (-10.0793, 36.9105) (-10.1526, 36.5672) (-10.358, 36.3089) (-10.5105, 36.2147) knots 0 0 0 1 2 3 3 3
  spline S193 degree 2 poles (-10.5105, 36.2147) (-10.6202, 36.1448) (-10.8556, 36.0391) knots 0 0 0 1 1 1
  spline S194 degree 2 poles (-10.8556, 36.0391) (-11.335, 35.828) (-11.5446, 35.6744) knots 0 0 0 1 1 1
  spline S195 degree 2 poles (-11.5446, 35.6744) (-11.5214, 35.5894) (-11.5143, 35.5665) knots 0 0 0 1 1 1
  spline S196 degree 2 poles (-11.5143, 35.5665) (-11.4369, 35.314) (-11.2883, 35.2479) knots 0 0 0 1 1 1
  spline S197 degree 2 poles (-11.2883, 35.2479) (-11.0897, 35.1554) (-10.7786, 35.2508) knots 0 0 0 1 1 1
  spline S198 degree 2 poles (-10.7786, 35.2508) (-10.4904, 35.3391) (-10.2775, 35.6276) (-10.2901, 35.9056) knots 0 0 0 1 2 2 2
  line L120 (-10.2901, 35.9056) -> (-9.8707, 35.9756)
  spline S199 degree 2 poles (-9.8707, 35.9756) (-9.8453, 35.7015) (-10.0001, 35.3053) (-10.4221, 34.989) (-10.7332, 34.8936) knots 0 0 0 1 2 3 3 3
  spline S200 degree 2 poles (-10.7332, 34.8936) (-11.0444, 34.7982) (-11.4766, 34.8247) (-11.7283, 34.9903) (-11.8156, 35.1477) knots 0 0 0 1 2 3 3 3
  spline S201 degree 2 poles (-11.8156, 35.1477) (-11.8689, 35.2485) (-11.9525, 35.5214) knots 0 0 0 1 1 1
  line L121 (-11.9525, 35.5214) -> (-12.1207, 36.0698)
  spline S202 degree 2 poles (-12.1207, 36.0698) (-12.2958, 36.6411) (-12.4424, 36.9282) (-12.562, 37.045) knots 0 0 0 1 2 2 2
  line L122 (-12.562, 37.045) -> (-12.1335, 37.1764)
  spline S203 degree 2 poles (-12.1335, 37.1764) (-12.0306, 37.0684) (-11.9604, 36.903) knots 0 0 0 1 1 1
  spline S204 degree 2 poles (-11.6457, 35.995) (-11.4494, 36.1556) (-11.0226, 36.3562) knots 0 0 0 1 1 1
  spline S205 degree 2 poles (-11.0226, 36.3562) (-10.7785, 36.4701) (-10.5975, 36.6261) (-10.5367, 36.8372) (-10.5696, 36.9444) knots 0 0 0 1 2 3 3 3
  spline S206 degree 2 poles (-10.5696, 36.9444) (-10.6196, 37.1076) (-10.9343, 37.2511) (-11.174, 37.1776) knots 0 0 0 1 2 2 2
  spline S207 degree 2 poles (-11.174, 37.1776) (-11.4112, 37.1048) (-11.7177, 36.7849) (-11.7489, 36.5772) knots 0 0 0 1 2 2 2
  spline S208 degree 2 poles (-11.7489, 36.5772) (-11.7722, 36.4166) (-11.6893, 36.1462) knots 0 0 0 1 1 1
  line L123 (-11.6893, 36.1462) -> (-11.6457, 35.995)
  line L124 (-13.0622, 36.8682) -> (-12.1519, 34.5002)
  line L125 (-12.1519, 34.5002) -> (-12.513, 34.3614)
  line L126 (-12.513, 34.3614) -> (-12.6422, 34.6975)
  spline S209 degree 2 poles (-12.6422, 34.6975) (-12.7543, 34.2086) (-13.2448, 34.02) knots 0 0 0 1 1 1
  spline S210 degree 2 poles (-13.2448, 34.02) (-13.459, 33.9377) (-13.8769, 33.9542) (-14.1519, 34.1343) (-14.2528, 34.2927) knots 0 0 0 1 2 3 3 3
  spline S211 degree 2 poles (-14.2528, 34.2927) (-14.3183, 34.3962) (-14.4255, 34.675) knots 0 0 0 1 1 1
  line L127 (-14.4255, 34.675) -> (-14.9845, 36.1292)
  line L128 (-14.9845, 36.1292) -> (-14.5836, 36.2833)
  line L129 (-14.5836, 36.2833) -> (-14.0304, 34.8441)
  spline S212 degree 2 poles (-14.0304, 34.8441) (-13.9365, 34.6001) (-13.7481, 34.3924) (-13.456, 34.3389) (-13.2942, 34.4011) knots 0 0 0 1 2 3 3 3
  spline S213 degree 2 poles (-13.2942, 34.4011) (-13.0377, 34.4997) (-12.7921, 34.9686) (-12.9663, 35.4217) knots 0 0 0 1 2 2 2
  line L130 (-12.9663, 35.4217) -> (-13.4631, 36.7141)
  line L131 (-13.4631, 36.7141) -> (-13.0622, 36.8682)
  line L132 (-15.5908, 35.8722) -> (-14.5182, 33.5731)
  line L133 (-14.5182, 33.5731) -> (-14.8688, 33.4095)
  line L134 (-14.8688, 33.4095) -> (-15.021, 33.7359)
  spline S214 degree 2 poles (-15.021, 33.7359) (-15.099, 33.2403) (-15.5752, 33.0182) knots 0 0 0 1 1 1
  spline S215 degree 2 poles (-15.5752, 33.0182) (-15.7831, 32.9212) (-16.2012, 32.9087) (-16.488, 33.0692) (-16.5997, 33.2202) knots 0 0 0 1 2 3 3 3
  spline S216 degree 2 poles (-16.5997, 33.2202) (-16.6722, 33.3189) (-16.7985, 33.5896) knots 0 0 0 1 1 1
  line L135 (-16.7985, 33.5896) -> (-17.4571, 35.0015)
  line L136 (-17.4571, 35.0015) -> (-17.0679, 35.1831)
  line L137 (-17.0679, 35.1831) -> (-16.416, 33.7857)
  spline S217 degree 2 poles (-16.416, 33.7857) (-16.3055, 33.5488) (-16.1031, 33.3547) (-15.808, 33.3217) (-15.6509, 33.395) knots 0 0 0 1 2 3 3 3
  spline S218 degree 2 poles (-15.6509, 33.395) (-15.4019, 33.5111) (-15.1894, 33.9959) (-15.3947, 34.4359) knots 0 0 0 1 2 2 2
  line L138 (-15.3947, 34.4359) -> (-15.98, 35.6906)
  line L139 (-15.98, 35.6906) -> (-15.5908, 35.8722)
  constraints: 2 other
extrude "Extrusion2" add sketch "Skizze2" along normal blind 1 contours L0 L1 S0 S1 S2 S3 S4 S5 S6 L2 L3 L4 | S11 S12 S13 S14 L6 L7 S15 S16 S17 L8 L9 S18 S19 | S24 L11 L12 S25 S26 S27 S28 S29 S30 S31 S32 S33 L13 L14 S34 S35 S36 S37 S38 S39 S40 | L15 L16 L17 L18 | L19 L20 L21 L22 | S41 S42 S43 S44 L23 S45 S46 S47 S48 S49 L24 L25 L26 S50 S51 L27 L28 | L30 L31 S56 S57 S58 L32 L33 L34 L35 L36 S59 S60 L37 | S61 S62 S63 S64 L38 L39 S65 S66 S67 L40 L41 S68 S69 | L43 L44 S74 S75 S76 S77 S78 S79 S80 L45 L46 L47 | S85 S86 L49 L50 L51 L52 L53 S87 S88 | L55 L56 L57 L58 L59 L60 L61 L62 | L63 L64 L65 S93 S94 L66 L67 L68 L69 L70 L71 L72 L73 L74 L75 | S95 S96 S97 S98 S99 S100 S101 S102 S103 L76 S104 S105 S106 L77 S107 L78 S108 | L80 L81 L82 L83 S114 S115 L84 L85 L86 L87 L88 L89 L90 L91 L92 | L93 S116 S117 S118 S119 S120 S121 S122 L94 S123 S124 S125 S126 S127 S128 S129 | L95 S130 S131 S132 S133 S134 L96 S135 S136 | L98 S140 S141 S142 S143 S144 S145 S146 S147 L99 S148 S149 S150 S151 S152 S153 S154 S155 | L100 S156 S157 S158 S159 S160 S161 S162 S163 L101 S164 S165 S166 S167 S168 S169 S170 S171 | L102 S172 S173 S174 S175 S176 L103 S177 S178 | L105 L106 L107 L108 | L109 L110 L111 S182 S183 S184 S185 L112 L113 L114 S186 S187 L115 L116 L117 S188 S189 L118 L119 | S190 S191 S192 S193 S194 S195 S196 S197 S198 L120 S199 S200 S201 L121 S202 L122 S203 | L124 L125 L126 S209 S210 S211 L127 L128 L129 S212 S213 L130 L131 | L132 L133 L134 S214 S215 S216 L135 L136 L137 S217 S218 L138 L139
